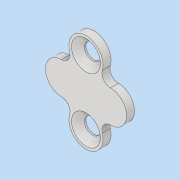
# Autodesk Inventor part: BearingRetentionBrace
Saved by Autodesk Inventor 2017 (Build 210142000, 142)
## iProperties
Created: 2017-10-02
Part Number: BearingRetentionBrace
Material: ABS Plastic
Document SubType Name: Modeling
Designer: Derek Wider
Density: 1.06 g/cm^3
Appearance: Smooth - White
Author: Derek Wider
Autodesk Inventor part; units mm, degrees
ref_plane "YZ Plane" through (0, 0, 0) normal (1, 0, 0) x (0, 1, 0)
ref_plane "XZ Plane" through (0, 0, 0) normal (0, 1, 0) x (-1, 0, 0)
ref_plane "XY Plane" through (0, 0, 0) normal (0, 0, 1) x (1, 0, 0)
sketch "Sketch1" plane through (0, 0, 0) normal (0, 0, 1) x (1, 0, 0)
  circle A0 centre (0, 0) radius 3.175
  circle A1 centre (9.652, 0) radius 3.175
  circle A2 centre (4.826, 6.35) radius 3.3655
  circle A3 centre (4.826, -6.35) radius 3.3655
  line L0 (4.826, 6.35) -> (0, 0) construction
  line L1 (0, 0) -> (4.826, -6.35) construction
  line L2 (4.826, -6.35) -> (9.652, 0) construction
  line L3 (9.652, 0) -> (4.826, 6.35) construction
  arc A4 (0, 3.175) -> (1.6102, 5.3573) centre (0, 4.8602) ccw
  arc A5 (1.6102, -5.3573) -> (0, -3.175) centre (0, -4.8602) ccw
  arc A6 (9.652, -3.175) -> (8.0418, -5.3573) centre (9.652, -4.8602) ccw
  arc A7 (8.0418, 5.3573) -> (9.652, 3.175) centre (9.652, 4.8602) ccw
  line L4 (0, 4.8602) -> (0, -4.8602) construction
  line L5 (9.652, 4.8602) -> (9.652, -4.8602) construction
  circle A8 centre (4.826, 6.35) radius 1.5875
  circle A9 centre (4.826, -6.35) radius 1.5875
  dimension "d0" = 6.35
  dimension "d1" = 9.652
  dimension "d2" = 12.7
  dimension "d3" = 6.731
  dimension "d4" = 3.175
  constraints: 16 point on circle, 12 end point, 10 centre point, 8 tangent, 5 vertical alignment, 4 equal length, 3 coincident, 3 equal radius, 2 vertical
  measures "d0" diameter of A0
  measures "d1" distance of L2.end point (0, 0)
  measures "d2" distance of L1.end L0.start
  measures "d3" diameter of A2
  measures "d4" diameter of A8
extrude "Extrusion1" add sketch "Sketch1" along normal blind 1.5875
chamfer "Chamfer1" distance 1.27 angle 45 2 edges at (3.2385, 6.35, 1.5875) (3.2385, -6.35, 1.5875)
body "Solid1"
